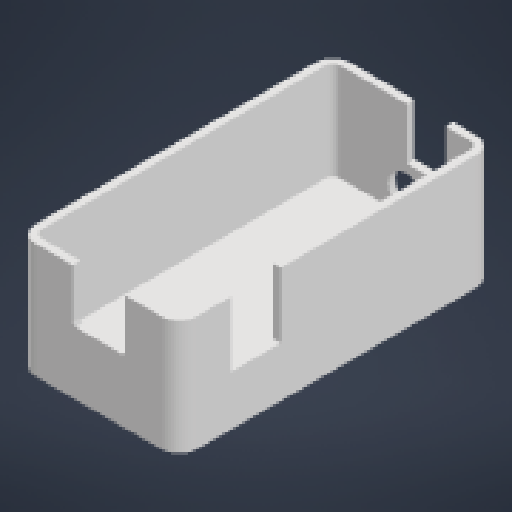
# Autodesk Inventor part: groundStation-top
Saved by Autodesk Inventor 2024 (Build 280153000, 153)
## iProperties
Created: 2024-02-06
Part Number: groundStation-top
Material: Generic
Document SubType Name: Modeling
Designer: madis
Density: 1 g/cm^3
Appearance: Default
Author: madis
Autodesk Inventor part; units mm, degrees
ref_plane "YZ Plane" through (0, 0, 0) normal (1, 0, 0) x (0, 1, 0)
ref_plane "XZ Plane" through (0, 0, 0) normal (0, 1, 0) x (-1, 0, 0)
ref_plane "XY Plane" through (0, 0, 0) normal (0, 0, 1) x (1, 0, 0)
sketch "Sketch1" plane through (0, 0, 0) normal (0, 1, 0) x (-1, 0, 0)
  line L0 (14.605, -25.4) -> (14.605, 25.4)
  line L1 (-14.605, -25.4) -> (-14.605, 25.4)
  line L2 (11.43, -28.575) -> (-11.43, -28.575)
  line L3 (11.43, 28.575) -> (-11.43, 28.575)
  arc A0 (11.43, -28.575) -> (14.605, -25.4) centre (11.43, -25.4) ccw
  arc A1 (-14.605, -25.4) -> (-11.43, -28.575) centre (-11.43, -25.4) ccw
  arc A2 (14.605, 25.4) -> (11.43, 28.575) centre (11.43, 25.4) ccw
  arc A3 (-11.43, 28.575) -> (-14.605, 25.4) centre (-11.43, 25.4) ccw
  point P0 (0, 0)
  dimension "d0" = 3.175
  dimension "d1" = 50.8
  dimension "d2" = 3.175
  dimension "d3" = 22.86
  dimension "d4" = 11.43
  dimension "d5" = 25.4
  dimension "d6" = 3.175
  dimension "d7" = 3.175
  constraints: 8 end point, 8 point on circle, 8 tangent, 4 centre point, 2 parallel, 1 horizontal, 1 vertical
  measures "d0" radius of A0
  measures "d1" distance of L0.start L0.end
  measures "d2" radius of A1
  measures "d3" distance of L2.start L2.end
  measures "d4" horizontal distance of point (0, 0) A0.centre
  measures "d5" vertical distance of point (0, 0) A0.centre
  measures "d6" radius of A2
  measures "d7" radius of A3
extrude "Extrusion1" add sketch "Sketch1" along normal blind 3.175
sketch "Sketch2" plane through (0, 3.175, 0) normal (0, 1, 0) x (1, 0, 0)
  line L0 (-13.208, 25.781) -> (-13.208, -25.781)
  line L1 (-14.605, 25.4) -> (-14.605, -25.4) projected
  arc A0 (-13.208, -25.781) -> (-11.811, -27.178) centre (-11.811, -25.781) ccw
  line L2 (-11.811, -27.178) -> (11.811, -27.178)
  line L3 (-11.43, -28.575) -> (11.43, -28.575) projected
  arc A1 (11.811, -27.178) -> (13.208, -25.781) centre (11.811, -25.781) ccw
  line L4 (13.208, -25.781) -> (13.208, 25.781)
  line L5 (14.605, -25.4) -> (14.605, 25.4) projected
  arc A2 (13.208, 25.781) -> (11.811, 27.178) centre (11.811, 25.781) ccw
  line L6 (11.811, 27.178) -> (-11.811, 27.178)
  arc A3 (-11.811, 27.178) -> (-13.208, 25.781) centre (-11.811, 25.781) ccw
  line L7 (-14.605, 25.4) -> (-14.605, -25.4) projected
  line L8 (-14.605, 25.4) -> (-14.605, -25.4)
  arc A4 (-14.605, -25.4) -> (-11.43, -28.575) centre (-11.43, -25.4) ccw projected
  arc A5 (-14.605, -25.4) -> (-11.43, -28.575) centre (-11.43, -25.4) ccw
  line L9 (-11.43, -28.575) -> (11.43, -28.575)
  arc A6 (11.43, -28.575) -> (14.605, -25.4) centre (11.43, -25.4) ccw projected
  arc A7 (11.43, -28.575) -> (14.605, -25.4) centre (11.43, -25.4) ccw
  line L10 (14.605, -25.4) -> (14.605, 25.4)
  arc A8 (14.605, 25.4) -> (11.43, 28.575) centre (11.43, 25.4) ccw projected
  line L11 (11.43, 28.575) -> (-11.43, 28.575)
  line L12 (-11.43, 28.575) -> (11.43, 28.575)
  arc A9 (-11.43, 28.575) -> (-14.605, 25.4) centre (-11.43, 25.4) ccw
  arc A10 (14.605, 25.4) -> (11.43, 28.575) centre (11.43, 25.4) ccw
  point P0 (0, 0)
  dimension "d10" = 1.397
  dimension "d11" = 1.397
  dimension "d12" = 1.397
  dimension "d14" = 1.397
  dimension "d15" = 1.397
  dimension "d16" = 1.397
  dimension "d17" = 1.397
  dimension "d18" = 1.397
  constraints: 18 end point, 17 point on circle, 13 tangent, 8 centre point, 4 vertical, 3 horizontal, 1 coincident, 1 collinear
  measures "d10" distance between parallel lines of L1 L0
  measures "d11" distance between parallel lines of L3 L2
  measures "d12" distance between parallel lines of L5 L4
  measures "d14" radius of A0
  measures "d15" radius of A1
  measures "d16" radius of A3
  measures "d17" radius of A2
  measures "d18" distance between parallel lines of L11 L6
extrude "Extrusion2" add sketch "Sketch2" along normal blind 17.78
sketch "Sketch4" plane through (-11.43, 0, 28.575) normal (0, 0, 1) x (1, 0, 0)
  line L0 (15.4305, 11.43) -> (7.4295, 11.43)
  line L1 (6.6675, 12.192) -> (6.6675, 20.955)
  line L2 (6.6675, 20.955) -> (16.1925, 20.955)
  line L3 (16.1925, 20.955) -> (16.1925, 12.192)
  line L4 (0, 20.955) -> (22.86, 20.955) projected
  line L5 (11.43, -2.422) -> (11.43, 18.2718) construction
  line L6 (22.86, 0) -> (22.86, 20.955) construction
  arc A0 (15.4019, 11.4305) -> (16.1925, 12.192) centre (15.4305, 12.192) ccw
  arc A1 (6.669, 12.2395) -> (7.4295, 11.43) centre (7.4295, 12.192) ccw
  point P0 (11.43, 0)
  dimension "d27" = 9.525
  dimension "d28" = 0
  dimension "d29" = 9.525
  dimension "d30" = 11.43
  dimension "d31" = 0.762
  dimension "d32" = 0.762
  constraints: 10 end point, 6 point on circle, 4 tangent, 2 centre point, 2 parallel, 1 horizontal, 1 perpendicular, 1 vertical, 1 other
  measures "d27" distance between parallel lines of L4 L0
  measures "d28" distance between parallel lines of L4 L2
  measures "d29" distance of L3.end L1.start
  measures "d30" distance between parallel lines of L6 L5
  measures "d31" radius of A0
  measures "d32" radius of A1
extrude "Extrusion3" cut sketch "Sketch4" against normal up to surface (1.397 mm away)
sketch "Sketch5" plane through (14.605, 0, 25.4) normal (1, 0, 0) x (0, 0, -1)
  line L0 (50.8, 20.955) -> (0, 20.955) projected
  line L1 (15.298, 9.091) -> (6.382, 9.091)
  line L2 (6.382, 9.091) -> (6.382, 20.955)
  line L3 (6.382, 20.955) -> (15.298, 20.955)
  line L4 (15.298, 20.955) -> (15.298, 9.091)
  line L5 (0, 0) -> (0, 20.955) projected
  line L6 (-3.175, 0) -> (-3.175, 20.955) projected
  point P0 (25.4, 0)
  point P1 (15.298, 20.955)
  dimension "d36" = 8.916
  dimension "d37" = 11.864
  dimension "d48" = 9.557
  constraints: 8 end point, 2 parallel, 1 horizontal, 1 perpendicular, 1 point on line
  measures "d36" distance of L1.start L1.end
  measures "d37" distance between parallel lines of L0 L1
  measures "d48" distance between parallel lines of L6 L2
extrude "Extrusion4" cut sketch "Sketch5" against normal up to surface (1.397 mm away)
sketch "Sketch6" plane through (11.43, 0, -28.575) normal (0, 0, -1) x (-1, 0, 0)
  line L0 (23.241, 20.955) -> (-0.381, 20.955) projected
  line L1 (11.128, 20.955) -> (4.112, 20.955)
  line L2 (4.112, 20.955) -> (4.112, 11.582)
  line L3 (4.112, 11.582) -> (11.128, 11.582)
  line L4 (11.128, 11.582) -> (11.128, 20.955)
  line L5 (0, 0) -> (0, 20.955) projected
  circle A0 centre (11.43, 6.8195) radius 3.175
  line L6 (22.86, 0) -> (22.86, 20.955) projected
  line L7 (-3.175, 0) -> (-3.175, 20.955) projected
  point P0 (11.43, 0)
  dimension "d41" = 7.016
  dimension "d42" = 9.373
  dimension "d45" = 6.35
  dimension "d46" = 4.7625
  dimension "d47" = 11.43
  dimension "d49" = 7.287
  constraints: 8 end point, 2 parallel, 1 centre point, 1 horizontal, 1 perpendicular, 1 point on line
  measures "d41" distance of L2.end L3.end
  measures "d42" distance between parallel lines of L0 L3
  measures "d45" diameter of A0
  measures "d46" distance from line of L3 A0.centre
  measures "d47" distance from line of L6 A0.centre
  measures "d49" distance between parallel lines of L7 L2
extrude "Extrusion5" cut sketch "Sketch6" against normal up to surface (1.397 mm away)
body "Solid1"
